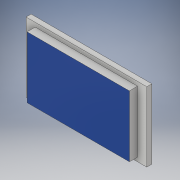
# Autodesk Inventor part: lcdsw
Saved by Autodesk Inventor 2019 (Build 230136000, 136)
## iProperties
Created: 2018-06-16
Part Number: lcdsw
Material: Generic
Document SubType Name: Modeling
Designer: daniel
Density: 1 g/cm^3
Appearance: Default
Author: daniel
Autodesk Inventor part; units mm, degrees
ref_plane "YZ Plane" through (0, 0, 0) normal (1, 0, 0) x (0, 1, 0)
ref_plane "XZ Plane" through (0, 0, 0) normal (0, 1, 0) x (-1, 0, 0)
ref_plane "XY Plane" through (0, 0, 0) normal (0, 0, 1) x (1, 0, 0)
sketch "Sketch1" plane through (0, 0, 0) normal (0, 0, 1) x (1, 0, 0)
  line L0 (-29.5, -17) -> (29.5, -17)
  line L1 (29.5, -17) -> (29.5, 17)
  line L2 (29.5, 17) -> (-29.5, 17)
  line L3 (-29.5, 17) -> (-29.5, -17)
  line L4 (-29.5, -17) -> (29.5, 17) construction
  line L5 (29.5, -17) -> (-29.5, 17) construction
  point P0 (0, 0)
  dimension "d0" = 59
  dimension "d1" = 34
  constraints: 12 end point, 2 midpoint, 2 parallel, 1 horizontal, 1 perpendicular
  measures "d0" distance of L2.end L1.end
  measures "d1" distance of L1.end L0.end
extrude "Extrusion1" add sketch "Sketch1" along normal blind 2.5
sketch "Sketch2" plane through (0, 0, 2.5) normal (0, 0, 1) x (1, 0, 0)
  line L0 (-25, -15) -> (25, -15)
  line L1 (25, -15) -> (25, 15)
  line L2 (25, 15) -> (-25, 15)
  line L3 (-25, 15) -> (-25, -15)
  line L4 (-25, -15) -> (25, 15) construction
  line L5 (25, -15) -> (-25, 15) construction
  point P0 (0, 0)
  dimension "d4" = 50
  dimension "d5" = 30
  constraints: 12 end point, 2 midpoint, 2 parallel, 1 horizontal, 1 perpendicular
  measures "d4" distance of L2.end L1.end
  measures "d5" distance of L1.end L0.end
extrude "Extrusion2" add sketch "Sketch2" along normal blind 4
sketch "Sketch3" plane through (0, 0, 0) normal (0, 0, -1) x (-1, 0, 0)
  line L0 (-41.3, 0) -> (41.3, 0) projected
  line L1 (27, 6) -> (19.5, 6)
  line L2 (19.5, 6) -> (19.5, -6)
  line L3 (19.5, -6) -> (27, -6)
  line L4 (27, -6) -> (27, 6)
  line L5 (27, 6) -> (19.5, -6) construction
  line L6 (19.5, 6) -> (27, -6) construction
  line L7 (29.5, 17) -> (29.5, -17) projected
  point P0 (0, 0)
  point P1 (23.25, 0)
  dimension "d8" = 7.5
  dimension "d9" = 12
  dimension "d10" = 2.5
  constraints: 12 end point, 2 midpoint, 2 parallel, 1 horizontal, 1 perpendicular, 1 point on line
  measures "d8" distance of L3.end L2.end
  measures "d9" distance of L2.end L1.end
  measures "d10" distance between parallel lines of L7 L4
extrude "Extrusion3" add sketch "Sketch3" along normal blind 5
body "Solid1"
